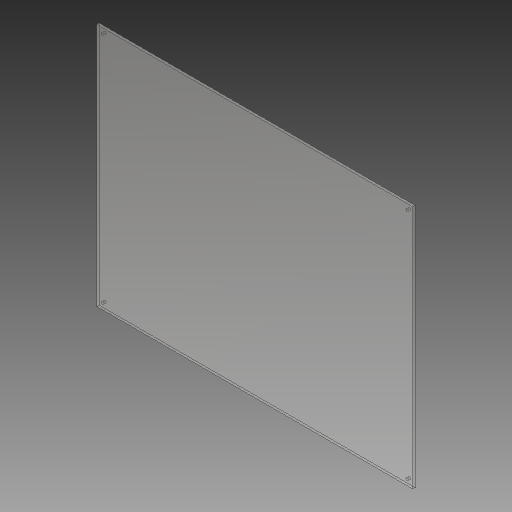
# Autodesk Inventor part: Plaque superieur
Saved by Autodesk Inventor 2017 (Build 210142000, 142)
## iProperties
Company: FABLAB Frenchmakers
Part Number: Plaque superieur
Project: 1400-PopCorn Machine
Material: Plastique PMMA
Catalog Web Link: http://www.frenchmakers.com/
Document SubType Name: Modeling
Designer: FABLAB Frenchmakers
Density: 1.188 g/cm^3
Appearance: Polycarbonate - Transparent
Stock Number: 1400-04-02
Mass: 444.179 g
Surface Area: 2536.59 cm^2
Volume: 373.888 cm^3
Author: Adrien MARY
Autodesk Inventor part; units mm, degrees
ref_plane "YZ Plane" through (0, 0, 0) normal (1, 0, 0) x (0, 1, 0)
ref_plane "XZ Plane" through (0, 0, 0) normal (0, 1, 0) x (-1, 0, 0)
ref_plane "XY Plane" through (0, 0, 0) normal (0, 0, 1) x (1, 0, 0)
sketch "Esquisse1" plane through (0, 0, 0) normal (0, 0, 1) x (1, 0, 0)
  line L0 (-200.75, -155.25) -> (200.75, -155.25)
  line L1 (200.75, -155.25) -> (200.75, 155.25)
  line L2 (200.75, 155.25) -> (-200.75, 155.25)
  line L3 (-200.75, 155.25) -> (-200.75, -155.25)
  line L4 (-200.75, -155.25) -> (200.75, 155.25) construction
  line L5 (200.75, -155.25) -> (-200.75, 155.25) construction
  point P0 (0, 0)
  dimension "Longueur_plaque_supérieur" = 401.5
  dimension "Profondeur_plaque_supérieur" = 310.5
  constraints: 12 end point, 2 midpoint, 2 parallel, 1 horizontal, 1 perpendicular
  measures "Longueur_plaque_supérieur" distance of L2.end L1.end
  measures "Profondeur_plaque_supérieur" distance of L2.end L0.start
extrude "Embase" add sketch "Esquisse1" along normal mid plane 3
sketch "Esquisse2" plane through (0, 0, 1.5) normal (0, 0, 1) x (1, 0, 0)
  line L0 (-200.75, 155.25) -> (-200.75, -155.25) construction
  line L1 (200.75, 155.25) -> (-200.75, 155.25) construction
  point P0 (0, 0)
  point P1 (-193.5, 148)
  dimension "d4" = 7.25
  dimension "d5" = 7.25
  measures "d4" distance from line of L0 point (-193.5, 148)
  measures "d5" distance from line of L1 point (-193.5, 148)
hole "Perçage" at (-193.5, 148, 1.5) direction (0, 0, -1) diameter 3.4 end through all clearance for "Vis à tête plate fraisée ISO 2009/7046" size "M3" standard "ISO"
mirror "Symétrie1" about plane through (0, 0, 0) normal (1, 0, 0) of "Perçage"
mirror "Symétrie2" about plane through (0, 0, 0) normal (0, 1, 0) of "Perçage", "Symétrie1"
